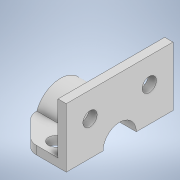
# Autodesk Inventor part: 2.6
Saved by Autodesk Inventor 2022 (Build 260153000, 153)
## iProperties
Created: 2023-04-17
Part Number: 2.6
Material: Genérico
Document SubType Name: Modeling
Designer: jpjoa
Density: 1 g/cm^3
Appearance: Padrão
Author: jpjoa
Autodesk Inventor part; units mm, degrees
ref_plane "YZ Plane" through (0, 0, 0) normal (1, 0, 0) x (0, 1, 0)
ref_plane "XZ Plane" through (0, 0, 0) normal (0, 1, 0) x (-1, 0, 0)
ref_plane "XY Plane" through (0, 0, 0) normal (0, 0, 1) x (1, 0, 0)
sketch "Esboço1" plane through (0, 0, 0) normal (0, 0, 1) x (1, 0, 0)
  line L0 (0, 0) -> (50, 0)
  line L1 (50, 0) -> (50, 50)
  line L2 (43, 50) -> (43, 7)
  line L3 (43, 7) -> (0, 7)
  line L4 (43, 50) -> (50, 50)
  line L5 (0, 7) -> (0, 0)
  dimension "d0" = 50
  dimension "d1" = 50
  dimension "d2" = 7
  constraints: 12 end point, 3 perpendicular, 2 horizontal, 1 other
  measures "d0" distance of L0.start L0.end
  measures "d1" distance of L0.end L1.end
  measures "d2" distance between parallel lines of L1 L2
extrude "Extrusão1" add sketch "Esboço1" along normal mid plane 90
sketch "Esboço2" plane through (43, 7, 45) normal (-1, 0, 0) x (0, 0, 1)
  arc A0 (-31, -7) -> (-59, -7) centre (-45, -7) ccw
  arc A1 (-24, -7) -> (-66, -7) centre (-45, -7) ccw
  line L0 (-90, -7) -> (0, -7) projected
  line L1 (-66, -7) -> (-24, -7)
  point P0 (-24, -7)
  point P1 (-66, -7)
  dimension "d5" = 28
  dimension "d6" = 42
  dimension "d7" = 42
  constraints: 4 point on circle, 3 coincident, 3 midpoint, 2 centre point, 2 end point, 2 point on line, 1 horizontal
  measures "d5" diameter of A0
  measures "d6" diameter of A1
  measures "d7" distance of L1.end L1.start
extrude "Extrusão2" cut sketch "Esboço2" along normal through all both and the other way through all contours L0 A0
extrude "Extrusão3" add sketch "Esboço2" along normal blind 43 contours A0 L0 A1
sketch "Esboço3" plane through (0, 7, 45) normal (0, 1, 0) x (1, 0, 0)
  circle A0 centre (30, 79) radius 6
  circle A1 centre (30, 11) radius 6
  line L0 (43, 0) -> (0, 0) projected
  line L1 (43, 90) -> (43, 0) projected
  point P0 (0, 45)
  dimension "d12" = 12
  dimension "d13" = 12
  dimension "d15" = 68
  dimension "d16" = 11
  dimension "d17" = 13
  constraints: 2 centre point, 1 vertical alignment
  measures "d12" diameter of A0
  measures "d13" diameter of A1
  measures "d15" distance of A0.centre A1.centre
  measures "d16" distance from line of L0 A1.centre
  measures "d17" distance from line of L1 A1.centre
extrude "Extrusão4" cut sketch "Esboço3" against normal through all
chamfer "Chanfro1" distance 20 angle 45 2 edges at (0, 3.5, 45) (0, 3.5, -45)
fillet "Arredondamento1" radius 11 4 edges at (0, 3.5, 25) (20, 3.5, 45) (0, 3.5, -25) (20, 3.5, -45)
sketch "Esboço4" plane through (43, 7, 45) normal (-1, 0, 0) x (0, 0, 1)
  circle A0 centre (-20, 22) radius 6
  circle A1 centre (-70, 22) radius 6
  line L0 (-3.2218, 0) -> (-16.7782, 0) projected
  line L1 (0, 43) -> (0, 0) projected
  line L2 (-90, 0) -> (-90, 43) projected
  point P0 (-45, -7)
  dimension "d24" = 12
  dimension "d25" = 12
  dimension "d26" = 50
  dimension "d27" = 22
  dimension "d28" = 20
  constraints: 2 centre point, 1 horizontal alignment
  measures "d24" diameter of A0
  measures "d25" diameter of A1
  measures "d26" distance of A0.centre A1.centre
  measures "d27" distance from line of L0 A0.centre
  measures "d28" distance from line of L1 A0.centre
extrude "Extrusão5" cut sketch "Esboço4" against normal through all
